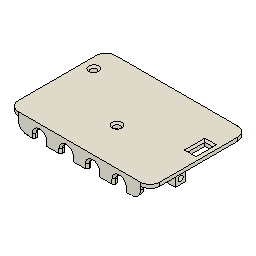
transmitter_assembly (Autodesk Fusion 360 archive; units mm, degrees)
design "transmitter_top_cover"
Autodesk Fusion 360 part; units mm, degrees
note: some values were not read from the file. Chosen so that the rebuilt part matches the saved one: which face or edge a step refers to. Set by a fixed rule: which sketch regions a step uses.
imported_body "Derived Base Feature1" makes body 1 makes body 2
imported_body "Derived Base Feature2" makes body 3 makes body 4
imported_body "Derived Base Feature3" makes body 5
imported_body "Derived Base Feature4" makes body 6
imported_body "Derived Base Feature5" makes body 7
imported_body "Derived Base Feature6" makes body 8
imported_body "Derived Base Feature7" makes body 9
imported_body "Derived Base Feature8" makes body 10
imported_body "Derived Base Feature9" makes body 11
imported_body "Derived Base Feature10" makes body 12
imported_body "Derived Base Feature11" makes body 13
imported_body "Derived Base Feature12" makes body 14
imported_body "Derived Base Feature13" makes body 15
sketch "Sketch1" plane through (0, 0, 0) normal (0, 1, 0) x (1, 0, 0)
  line L0 (34.5, 27.5) -> (-34.5, 27.5)
  line L1 (-40, 22) -> (-40, -22)
  line L2 (-34.5, -27.5) -> (34.5, -27.5)
  line L3 (40, -22) -> (40, 22)
  line L4 (40, 27.5) -> (-40, -27.5) construction
  line L5 (-40, 27.5) -> (40, -27.5) construction
  arc A0 (-34.5, 27.5) -> (-40, 22) centre (-34.5, 22) ccw
  arc A1 (40, 22) -> (34.5, 27.5) centre (34.5, 22) ccw
  arc A2 (34.5, -27.5) -> (40, -22) centre (34.5, -22) ccw
  arc A3 (-40, -22) -> (-34.5, -27.5) centre (-34.5, -22) ccw
  dimension "d1" = 80
  dimension "d2" = 55
  dimension "d3" = 5.5
  constraint horizontal L0
  constraint perpendicular L0 L1
  constraint parallel L0 L2
  constraint parallel L1 L3
  constraint coincident L4 origin
  constraint coincident L5 origin
  constraint coincident L5.start L1
  constraint coincident L5.start L0
  constraint tangent L1 A0
  constraint tangent L0 A0
  constraint coincident L4.start L0
  constraint coincident L4.start L3
  constraint tangent L0 A1
  constraint tangent L3 A1
  constraint coincident L5.end L3
  constraint coincident L5.end L2
  constraint tangent L3 A2
  constraint tangent L2 A2
  constraint equal A1 A2
  constraint coincident L4.end L2
  constraint coincident L4.end L1
  constraint tangent L2 A3
  constraint tangent L1 A3
  constraint equal A1 A3
  constraint equal A0 A1
  measures "d1" distance of L4.end L5.end
  measures "d2" distance of L5.start L4.end
  measures "d3" radius of A0
extrude "Extrude1" add sketch "Sketch1" against normal blind 2 separate body makes body 16
sketch "Sketch2" plane through (0, -2, 0) normal (0, -1, 0) x (1, 0, 0)
  arc A0 (-34.5, 27.5) -> (-40, 22) centre (-34.5, 22) ccw
  line L0 (-40, 22) -> (-40, -22)
  arc A1 (-40, -22) -> (-34.5, -27.5) centre (-34.5, -22) ccw
  line L1 (-34.5, -27.5) -> (34.5, -27.5)
  arc A2 (34.5, -27.5) -> (40, -22) centre (34.5, -22) ccw
  line L2 (40, -22) -> (40, 22)
  arc A3 (40, 22) -> (34.5, 27.5) centre (34.5, 22) ccw
  line L3 (34.5, 27.5) -> (-34.5, 27.5)
  line L4 (34.5, 25.5) -> (-34.5, 25.5)
  line L5 (-38, 22) -> (-38, -22)
  line L6 (-34.5, -25.5) -> (34.5, -25.5)
  line L7 (38, -22) -> (38, 22)
  line L8 (38, 25.5) -> (-38, -25.5) construction
  line L9 (-38, 25.5) -> (38, -25.5) construction
  arc A4 (-34.5, 25.5) -> (-38, 22) centre (-34.5, 22) ccw
  arc A5 (38, 22) -> (34.5, 25.5) centre (34.5, 22) ccw
  arc A6 (34.5, -25.5) -> (38, -22) centre (34.5, -22) ccw
  arc A7 (-38, -22) -> (-34.5, -25.5) centre (-34.5, -22) ccw
  dimension "d7" = 76
  dimension "d8" = 51
  dimension "d9" = 3.5
  constraint horizontal L4
  constraint perpendicular L4 L5
  constraint parallel L4 L6
  constraint parallel L5 L7
  constraint coincident L8 origin
  constraint coincident L9 origin
  constraint coincident L9.start L5
  constraint coincident L9.start L4
  constraint tangent L5 A4
  constraint tangent L4 A4
  constraint coincident L8.start L4
  constraint coincident L8.start L7
  constraint tangent L4 A5
  constraint tangent L7 A5
  constraint coincident L9.end L7
  constraint coincident L9.end L6
  constraint tangent L7 A6
  constraint tangent L6 A6
  constraint equal A5 A6
  constraint coincident L8.end L6
  constraint coincident L8.end L5
  constraint tangent L6 A7
  constraint tangent L5 A7
  constraint equal A5 A7
  constraint equal A4 A5
  measures "d7" distance of L8.end L9.end
  measures "d8" distance of L9.start L8.end
  measures "d9" radius of A4
extrude "Extrude2" add sketch "Sketch2" along normal blind 1 contours L4 L5 L6 L7 A4 A5 A6 A7 bodies 16
sketch "Sketch3" plane through (0, 0, -27.5) normal (0, 0, -1) x (-1, 0, 0)
  line L0 (34.5, 0) -> (-34.5, 0)
  line L1 (-34.5, 0) -> (-34.5, -2)
  line L2 (-34.5, -2) -> (34.5, -2)
  line L3 (34.5, -2) -> (34.5, 0)
  line L4 (-34.5, 0) -> (34.5, 0)
  line L5 (34.5, 0) -> (34.5, -4)
  line L6 (29.5, -9) -> (-29.5, -9)
  line L7 (-34.5, -4) -> (-34.5, 0)
  arc A0 (29.5, -9) -> (34.5, -4) centre (29.5, -4) ccw
  arc A1 (-34.5, -4) -> (-29.5, -9) centre (-29.5, -4) ccw
  point P0 (-34.5, -9)
  dimension "d13" = 9
  dimension "d14" = 5
  constraint horizontal L4
  constraint vertical L5
  constraint horizontal L6
  constraint vertical L7
  constraint coincident L0.end L1.start
  constraint coincident L0.start L3.end
  constraint tangent L5 A0
  constraint tangent L6 A0
  constraint coincident P0 L6
  constraint coincident P0 L7
  constraint tangent L6 A1
  constraint tangent L7 A1
  constraint equal A0 A1
  measures "d13" distance of L0.end P0
  measures "d14" radius of A0
extrude "Extrude3" add sketch "Sketch3" against normal blind 2 bodies 16
mirror "Mirror1" about plane through (0, 0, 0) normal (0, 0, 1) of "Extrude3"
sketch "Sketch4" plane through (0, 0, -27.5) normal (0, 0, -1) x (-1, 0, 0)
  line L0 (34.5, 0) -> (-34.5, 0)
  line L1 (-34.5, 0) -> (-34.5, -2)
  line L2 (-34.5, -2) -> (-34.5, -4)
  arc A0 (-34.5, -4) -> (-29.5, -9) centre (-29.5, -4) ccw
  line L3 (-29.5, -9) -> (29.5, -9)
  arc A1 (29.5, -9) -> (34.5, -4) centre (29.5, -4) ccw
  line L4 (34.5, -4) -> (34.5, -2)
  line L5 (34.5, -2) -> (34.5, 0)
  line L6 (24.8, -5.105) -> (20.2, -5.105)
  line L7 (20.2, -5.105) -> (20.2, -9)
  line L8 (20.2, -9) -> (24.8, -9)
  line L9 (24.8, -9) -> (24.8, -5.105)
  line L10 (5.03, -9) -> (13.97, -9)
  line L11 (13.97, -9) -> (13.97, -7.23)
  line L12 (12.69, -5.95) -> (6.31, -5.95)
  line L13 (5.03, -7.23) -> (5.03, -9)
  line L14 (5.03, -9) -> (13.97, -5.95) construction
  line L15 (13.97, -9) -> (5.03, -5.95) construction
  arc A2 (13.97, -7.23) -> (12.69, -5.95) centre (12.69, -7.23) ccw
  arc A3 (6.31, -5.95) -> (5.03, -7.23) centre (6.31, -7.23) ccw
  line L16 (0, -9) -> (37.5, -9) construction
  line L17 (24.8, -9) -> (20.2, -5.105) construction
  line L18 (20.2, -9) -> (24.8, -5.105) construction
  point P0 (9.5, -7.475)
  point P1 (22.5, -7.0525)
  dimension "d83" = 8.94
  dimension "d84" = 3.05
  dimension "d85" = 1.28
  dimension "d87" = 4.6
  dimension "d88" = 3.895
  dimension "d119" = 37.5
  dimension "d120" = 28
  dimension "d121" = 15
  constraint horizontal L6
  constraint vertical L7
  constraint horizontal L8
  constraint vertical L9
  constraint coincident L3 L7.end
  constraint horizontal L10
  constraint perpendicular L10 L11
  constraint parallel L10 L12
  constraint parallel L11 L13
  constraint coincident L14 P0
  constraint coincident L15 P0
  constraint coincident L14.end L12
  constraint coincident L14.end L11
  constraint tangent L12 A2
  constraint tangent L11 A2
  constraint coincident L15.end L13
  constraint coincident L15.end L12
  constraint tangent L13 A3
  constraint tangent L12 A3
  constraint equal A2 A3
  constraint coincident L3 L10.end
  constraint midpoint L3 L16.start
  constraint perpendicular L13 L16
  constraint coincident L18 P1
  constraint coincident L17 P1
  measures "d83" distance of L14.end L15.end
  measures "d84" distance of L10.end L14.end
  measures "d85" radius of A2
  measures "d87" distance of L6.start L6.end
  measures "d88" distance of L6.start L8.end
  measures "d119" distance of L16.start L16.end
  measures "d120" horizontal distance of P0 L16.end
  measures "d121" horizontal distance of L16.end P1
extrude "Extrude4" cut sketch "Sketch4" against normal up to surface (2 mm away) contours L3 L6 L7 L8 L9 | L3 L10 L11 L12 L13 A2 A3 bodies 16
sketch "Sketch10" plane through (0, 0, 27.5) normal (0, 0, 1) x (1, 0, 0)
  line L0 (34.5, 0) -> (-34.5, 0)
  line L1 (-34.5, 0) -> (-34.5, -2)
  line L2 (-34.5, -2) -> (-34.5, -4)
  arc A0 (-34.5, -4) -> (-29.5, -9) centre (-29.5, -4) ccw
  line L3 (-29.5, -9) -> (29.5, -9)
  arc A1 (29.5, -9) -> (34.5, -4) centre (29.5, -4) ccw
  line L4 (34.5, -4) -> (34.5, -2)
  line L5 (34.5, -2) -> (34.5, 0)
  circle A2 centre (-22.5, -6.5) radius 3.05
  circle A3 centre (-7.5, -6.5) radius 3.05
  circle A4 centre (7.5, -6.5) radius 3.05
  circle A5 centre (22.5, -6.5) radius 3.05
  line L6 (-22.5, -6.5) -> (22.5, -6.5) construction
  line L7 (0, 0) -> (0, -9) construction
  line L8 (-25.55, -6.5) -> (-25.55, -9)
  line L9 (-19.45, -6.5) -> (-19.45, -9)
  line L10 (-10.55, -6.5) -> (-10.55, -9)
  line L11 (-4.45, -6.5) -> (-4.45, -9)
  line L12 (4.45, -6.5) -> (4.45, -9)
  line L13 (10.55, -6.5) -> (10.55, -9)
  line L14 (19.45, -6.5) -> (19.45, -9)
  line L15 (25.55, -6.5) -> (25.55, -9)
  point P0 (0, -6.5)
  dimension "d92" = 15
  dimension "d93" = 0
  dimension "d96" = 6.1
  dimension "d97" = 2.5
  constraint coincident A2.centre L6.start
  constraint coincident A5.centre L6.end
  constraint coincident L7.start origin
  constraint midpoint L3 L7.end
  constraint midpoint L6 P0
  constraint coincident L7 P0
  constraint coincident A2 L8.start
  constraint coincident L3 L8.end
  constraint perpendicular L3 L8
  constraint tangent A2 L8
  constraint coincident A2 L9.start
  constraint coincident L3 L9.end
  constraint perpendicular L3 L9
  constraint tangent A2 L9
  measures "d96" diameter of A2
  measures "d97" distance of L3 A2.centre
extrude "Extrude10" cut sketch "Sketch10" against normal blind 2 contours L3 A5 L15 | L3 A2 L8 | L3 A5 | L3 A2 | L3 A5 L14 | L3 A2 L9 | L3 A4 L13 | L3 A3 L10 | L3 A4 | L3 A3 | L3 A4 L12 | L3 A3 L11 picked at (23.3012, -7.8261) picked at (-23.3086, -6.3422) picked at (8.1001, -5.2539) picked at (-7.5633, -5.6506) bodies 16
sketch "Sketch5" plane through (0, 0, 0) normal (0, 1, 0) x (-1, 0, 0)
  arc A0 (34.5, -27.5) -> (40, -22) centre (34.5, -22) ccw
  line L0 (40, -22) -> (40, 22)
  arc A1 (40, 22) -> (34.5, 27.5) centre (34.5, 22) ccw
  line L1 (34.5, 27.5) -> (-34.5, 27.5)
  arc A2 (-34.5, 27.5) -> (-40, 22) centre (-34.5, 22) ccw
  line L2 (-40, 22) -> (-40, -22)
  arc A3 (-40, -22) -> (-34.5, -27.5) centre (-34.5, -22) ccw
  line L3 (-34.5, -27.5) -> (34.5, -27.5)
  circle A4 centre (42.5, -18) radius 1.5
  circle A5 centre (42.5, -18) radius 1.5
  circle A6 centre (40, 15.27) radius 1.5
  circle A7 centre (30, 15.27) radius 1.5
  circle A8 centre (20, 15.27) radius 1.5
  circle A9 centre (10, 15.27) radius 1.5
  circle A10 centre (-10, 15.27) radius 1.5
  circle A11 centre (-20, 15.27) radius 1.5
  circle A12 centre (-40, 15.27) radius 1.5
  circle A13 centre (-30, 15.27) radius 1.5
  line L4 (-48.016, -4.69) -> (-48.27, -4.944)
  line L5 (-48.27, -4.944) -> (-48.27, -6.976)
  line L6 (-48.27, -6.976) -> (-48.016, -7.23)
  line L7 (-48.016, -7.23) -> (-48.27, -7.484)
  line L8 (-48.27, -7.484) -> (-48.27, -9.516)
  line L9 (-48.27, -9.516) -> (-48.016, -9.77)
  line L10 (-48.016, -9.77) -> (-48.27, -10.024)
  line L11 (-48.27, -10.024) -> (-48.27, -12.056)
  line L12 (-48.27, -12.056) -> (-48.016, -12.31)
  line L13 (-48.016, -12.31) -> (-45.984, -12.31)
  line L14 (-45.984, -12.31) -> (-45.73, -12.056)
  line L15 (-45.73, -12.056) -> (-45.73, -10.024)
  line L16 (-45.73, -10.024) -> (-45.984, -9.77)
  line L17 (-45.984, -9.77) -> (-45.73, -9.516)
  line L18 (-45.73, -9.516) -> (-45.73, -7.484)
  line L19 (-45.73, -7.484) -> (-45.984, -7.23)
  line L20 (-45.984, -7.23) -> (-45.73, -6.976)
  line L21 (-45.73, -6.976) -> (-45.73, -4.944)
  line L22 (-45.73, -4.944) -> (-45.984, -4.69)
  line L23 (-45.984, -4.69) -> (-48.016, -4.69)
  line L24 (-46.68, -5.64) -> (-46.68, -6.28)
  line L25 (-46.68, -6.28) -> (-47.32, -6.28)
  line L26 (-47.32, -6.28) -> (-47.32, -5.64)
  line L27 (-47.32, -5.64) -> (-46.68, -5.64)
  line L28 (-46.68, -8.82) -> (-47.32, -8.82)
  line L29 (-47.32, -8.82) -> (-47.32, -8.18)
  line L30 (-47.32, -8.18) -> (-46.68, -8.18)
  line L31 (-46.68, -8.18) -> (-46.68, -8.82)
  line L32 (-47.32, -10.72) -> (-46.68, -10.72)
  line L33 (-46.68, -10.72) -> (-46.68, -11.36)
  line L34 (-46.68, -11.36) -> (-47.32, -11.36)
  line L35 (-47.32, -11.36) -> (-47.32, -10.72)
  line L36 (-49.27, -13.31) -> (-44.73, -13.31)
  line L37 (-44.73, -13.31) -> (-44.73, -3.69)
  line L38 (-44.73, -3.69) -> (-49.27, -3.69)
  line L39 (-49.27, -3.69) -> (-49.27, -13.31)
  line L40 (-49.27, -13.31) -> (-44.73, -3.69) construction
  line L41 (-44.73, -13.31) -> (-49.27, -3.69) construction
  circle A14 centre (-40, 15.27) radius 1.75
  circle A15 centre (-30, 15.27) radius 1.75
  circle A16 centre (-20, 15.27) radius 1.75
  circle A17 centre (-10, 15.27) radius 1.75
  circle A18 centre (10, 15.27) radius 1.75
  circle A19 centre (20, 15.27) radius 1.75
  circle A20 centre (30, 15.27) radius 1.75
  circle A21 centre (40, 15.27) radius 1.75
  point P0 (-47, -8.5)
  dimension "d22" = 1
  dimension "d23" = 1
  dimension "d24" = 1
  dimension "d25" = 1
  dimension "d69" = 0.25
  dimension "d72" = 80
  dimension "d73" = 0
  constraint horizontal L36
  constraint perpendicular L36 L37
  constraint parallel L36 L38
  constraint parallel L37 L39
  constraint coincident L40 P0
  constraint coincident L41 P0
  measures "d22" distance of L13 L36
  measures "d23" distance of L15 L37
  measures "d24" distance of L23 L38
  measures "d25" distance of L8 L39
extrude "Extrude5" [suppressed]
sketch "Sketch6" plane through (0, -3, 0) normal (0, -1, 0) x (1, 0, 0)
  arc A0 (-38, -22) -> (-34.5, -25.5) centre (-34.5, -22) ccw
  line L0 (-34.5, -25.5) -> (34.5, -25.5)
  arc A1 (34.5, -25.5) -> (38, -22) centre (34.5, -22) ccw
  line L1 (38, -22) -> (38, 22)
  arc A2 (38, 22) -> (34.5, 25.5) centre (34.5, 22) ccw
  line L2 (34.5, 25.5) -> (-34.5, 25.5)
  arc A3 (-34.5, 25.5) -> (-38, 22) centre (-34.5, 22) ccw
  line L3 (-38, 22) -> (-38, -22)
  circle A4 centre (-40, 15.27) radius 2.5
  circle A5 centre (-30, 15.27) radius 2.5
  circle A6 centre (-20, 15.27) radius 2.5
  circle A7 centre (-10, 15.27) radius 2.5
  circle A8 centre (10, 15.27) radius 2.5
  circle A9 centre (20, 15.27) radius 2.5
  circle A10 centre (30, 15.27) radius 2.5
  circle A11 centre (40, 15.27) radius 2.5
  circle A12 centre (-42.5, -18) radius 2.5
  circle A13 centre (-40, 15.27) radius 3.5
  circle A14 centre (-30, 15.27) radius 3.5
  circle A15 centre (-20, 15.27) radius 3.5
  circle A16 centre (-10, 15.27) radius 3.5
  circle A17 centre (10, 15.27) radius 3.5
  circle A18 centre (20, 15.27) radius 3.5
  circle A19 centre (30, 15.27) radius 3.5
  circle A20 centre (40, 15.27) radius 3.5
  circle A21 centre (-42.5, -18) radius 3
  circle A22 centre (-10, 15.27) radius 1.75
  circle A23 centre (10, 15.27) radius 1.75
  circle A24 centre (-20, 15.27) radius 1.75
  circle A25 centre (20, 15.27) radius 1.75
  circle A26 centre (30, 15.27) radius 1.75
  circle A27 centre (-30, 15.27) radius 1.75
  dimension "d35" = 5
  dimension "d36" = 5
  dimension "d44" = 7
  dimension "d45" = 6
  constraint concentric A4 A13
  constraint concentric A5 A14
  constraint concentric A6 A15
  constraint concentric A7 A16
  constraint concentric A8 A17
  constraint concentric A9 A18
  constraint concentric A11 A20
  constraint concentric A12 A21
  constraint equal A10 A11
  constraint equal A9 A10
  constraint equal A8 A9
  constraint equal A7 A8
  constraint equal A6 A7
  constraint equal A5 A6
  constraint equal A4 A5
  constraint equal A19 A20
  constraint equal A18 A19
  constraint equal A17 A18
  constraint equal A16 A17
  constraint equal A15 A16
  constraint equal A14 A15
  constraint equal A13 A14
  measures "d35" diameter of A11
  measures "d36" diameter of A12
  measures "d44" diameter of A20
  measures "d45" diameter of A21
extrude "Extrude6" [suppressed]
sketch "Sketch7" plane through (38, 0, 0) normal (1, 0, 0) x (0, 0, -1)
  line L0 (-22, -2) -> (-22, -3)
  line L1 (-22, -3) -> (22, -3)
  line L2 (22, -3) -> (22, -2)
  line L3 (22, -8.99) -> (-22, -8.99)
  line L4 (-11.225, -3) -> (-5.225, -3)
  line L5 (-5.225, -3) -> (-5.225, -8.99)
  line L6 (-5.225, -8.99) -> (-11.225, -8.99)
  line L7 (-11.225, -8.99) -> (-11.225, -3)
  circle A0 centre (-8.225, -5.995) radius 1.45
  line L8 (22, -2) -> (-22, -2)
  dimension "d48" = 6
  dimension "d49" = 10.775
  dimension "d60" = 2.9
  dimension "d61" = 2.995
  dimension "d62" = 13.775
  constraint horizontal L4
  constraint vertical L5
  constraint horizontal L6
  constraint vertical L7
  constraint coincident L3 L5.end
  constraint coincident L1 L4.start
  measures "d48" distance of L4.start L4.end
  measures "d49" distance of L3.end L7
  measures "d60" diameter of A0
  measures "d61" distance of L3 A0.centre
  measures "d62" horizontal distance of L3.end A0.centre
extrude "Extrude7" add sketch "Sketch7" against normal blind 5 contours L1 L3 L4 L5 L6 L7 bodies 16
sketch "Sketch8" plane through (0, 0, 25.5) normal (0, 0, 1) x (1, 0, 0)
  line L0 (34.5, -2) -> (-34.5, -2)
  line L1 (-34.5, -2) -> (-34.5, -3)
  line L2 (-34.5, -3) -> (34.5, -3)
  line L3 (34.5, -3) -> (34.5, -2)
  line L4 (47, -8.99) -> (-47, -8.99)
  line L5 (-3, -3) -> (3, -3)
  line L6 (3, -3) -> (3, -8.99)
  line L7 (3, -8.99) -> (-3, -8.99)
  line L8 (-3, -8.99) -> (-3, -3)
  circle A0 centre (12.5, -5.995) radius 1.45
  dimension "d52" = 6
  dimension "d53" = 44
  dimension "d63" = 2.9
  dimension "d64" = 47
  dimension "d65" = 2.995
  constraint horizontal L5
  constraint vertical L6
  constraint horizontal L7
  constraint vertical L8
  constraint coincident L2 L5.start
  constraint coincident L4 L6.end
  measures "d52" distance of L5.start L5.end
  measures "d53" distance of L4.end L7.end
  measures "d63" diameter of A0
  measures "d64" distance of L1 A0.centre
  measures "d65" distance of L7 A0.centre
extrude "Extrude8" [suppressed]
sketch "Sketch9" plane through (-38, 0, 0) normal (-1, 0, 0) x (0, 0, 1)
  line L0 (-22, -2) -> (-22, -3)
  line L1 (-22, -3) -> (22, -3)
  line L2 (22, -3) -> (22, -2)
  line L3 (-12, -3) -> (-6, -3)
  line L4 (-6, -3) -> (-6, -8.99)
  line L5 (-6, -8.99) -> (-12, -8.99)
  line L6 (-12, -8.99) -> (-12, -3)
  line L7 (22, -8.99) -> (-22, -8.99)
  circle A0 centre (-9, -5.995) radius 1.45
  line L8 (22, -2) -> (-22, -2)
  dimension "d56" = 6
  dimension "d57" = 10
  dimension "d66" = 2.9
  dimension "d67" = 2.995
  dimension "d68" = 13
  constraint horizontal L3
  constraint vertical L4
  constraint horizontal L5
  constraint vertical L6
  constraint coincident L1 L3.start
  constraint coincident L4.end L7
  measures "d56" distance of L4.end L5.end
  measures "d57" distance of L5.end L7.end
  measures "d66" diameter of A0
  measures "d67" distance of L7 A0.centre
  measures "d68" horizontal distance of L7.end A0.centre
extrude "Extrude9" add sketch "Sketch9" against normal blind 5 contours L1 L3 L4 L5 L6 L7 bodies 16
chamfer "Chamfer1" [suppressed]
chamfer "Chamfer2" distance 1 angle 45 3 edges at (-24.8, -7.0525, -27.5) (-22.5, -5.105, -27.5) (-20.2, -7.0525, -27.5) on bodies 16
chamfer "Chamfer2" distance 1 angle 45 5 edges at (-9.5, -5.95, -27.5) (-5.4049, -6.3249, -27.5) (-5.03, -8.115, -27.5) (-13.97, -8.115, -27.5) (-13.5951, -6.3249, -27.5) on bodies 16
chamfer "Chamfer2" distance 1 angle 45 12 edges at (-22.5, -3.45, 27.5) (-19.45, -7.75, 27.5) (-25.55, -7.75, 27.5) (-7.5, -3.45, 27.5) (-4.45, -7.75, 27.5) (-10.55, -7.75, 27.5) (10.55, -7.75, 27.5) (4.45, -7.75, 27.5) (7.5, -3.45, 27.5) (22.5, -3.45, 27.5) (25.55, -7.75, 27.5) (19.45, -7.75, 27.5) on bodies 16
fillet "Fillet1" [suppressed]
sketch "Sketch11" plane through (0, -3, 0) normal (0, -1, 0) x (1, 0, 0)
  line L0 (-33, -12) -> (-38, -12)
  line L1 (-38, -12) -> (-38, -22)
  arc A0 (-38, -22) -> (-34.5, -25.5) centre (-34.5, -22) ccw
  line L2 (-34.5, -25.5) -> (34.5, -25.5)
  arc A1 (34.5, -25.5) -> (38, -22) centre (34.5, -22) ccw
  line L3 (38, -22) -> (38, 5.225)
  line L4 (38, 5.225) -> (33, 5.225)
  line L5 (33, 5.225) -> (33, 11.225)
  line L6 (33, 11.225) -> (38, 11.225)
  line L7 (38, 11.225) -> (38, 22)
  arc A2 (38, 22) -> (34.5, 25.5) centre (34.5, 22) ccw
  line L8 (34.5, 25.5) -> (-34.5, 25.5)
  arc A3 (-34.5, 25.5) -> (-38, 22) centre (-34.5, 22) ccw
  line L9 (-38, 22) -> (-38, -6)
  line L10 (-38, -6) -> (-33, -6)
  line L11 (-33, -6) -> (-33, -12)
  line L12 (37.5, 25) -> (-37.5, 25) construction
  line L13 (-37.5, 25) -> (-37.5, -25) construction
  line L14 (-37.5, -25) -> (37.5, -25) construction
  line L15 (37.5, -25) -> (37.5, 25) construction
  line L16 (37.5, 25) -> (-37.5, -25) construction
  line L17 (-37.5, 25) -> (37.5, -25) construction
  circle A4 centre (0, 6.27) radius 1.75
  circle A5 centre (0, 6.27) radius 2.5
  circle A6 centre (0, 6.27) radius 3
  line L18 (32.23, -11.27) -> (36.77, -11.27)
  line L19 (36.77, -11.27) -> (36.77, -1.65)
  line L20 (36.77, -1.65) -> (32.23, -1.65)
  line L21 (32.23, -1.65) -> (32.23, -11.27)
  line L22 (32.23, -11.27) -> (36.77, -1.65) construction
  line L23 (36.77, -11.27) -> (32.23, -1.65) construction
  circle A7 centre (-34.23, -14.825) radius 1.75
  circle A8 centre (-34.23, -14.825) radius 2.5
  circle A9 centre (-34.23, -14.825) radius 3
  point P0 (34.5, -6.46)
  dimension "d99" = 75
  dimension "d100" = 50
  dimension "d101" = 37.5
  dimension "d103" = 18.73
  dimension "d104" = 3.5
  dimension "d107" = 5
  dimension "d108" = 6
  dimension "d114" = 3
  dimension "d115" = 18.54
  dimension "d116" = 4.54
  dimension "d117" = 9.62
  dimension "d123" = 3.5
  dimension "d124" = 5
  dimension "d125" = 6
  dimension "d126" = 3.27
  dimension "d131" = 10.175
  constraint horizontal L12
  constraint perpendicular L12 L13
  constraint parallel L12 L14
  constraint parallel L13 L15
  constraint coincident L16 origin
  constraint coincident L17 origin
  constraint concentric A4 A5
  constraint concentric A5 A6
  constraint horizontal L18
  constraint perpendicular L18 L19
  constraint parallel L18 L20
  constraint parallel L19 L21
  constraint coincident L22 P0
  constraint coincident L23 P0
  constraint concentric A7 A8
  constraint concentric A8 A9
  measures "d99" distance of L13.end L14.end
  measures "d100" distance of L12.end L13.end
  measures "d101" horizontal distance of L13.end A4.centre
  measures "d103" distance of L12 A4.centre
  measures "d104" diameter of A4
  measures "d107" diameter of A5
  measures "d108" diameter of A6
  measures "d114" distance of L15 P0
  measures "d115" distance of L14 P0
  measures "d116" distance of L18.start L18.end
  measures "d117" distance of L18.start L20.end
  measures "d123" diameter of A7
  measures "d124" diameter of A8
  measures "d125" diameter of A9
  measures "d126" horizontal distance of L12.end A7.centre
  measures "d131" vertical distance of L13.end A7.centre
extrude "Extrude11" cut sketch "Sketch11" against normal blind 3 contours A4 | L18 L19 L20 L21 | A7 bodies 16
extrude "Extrude12" add sketch "Sketch11" along normal blind 5.99 contours L0 A9 | L0 A9 | A6 bodies 16
chamfer "Chamfer3" distance 1 angle 45 1 edges at (-1.6316, 0, 5.6372) on bodies 16
chamfer "Chamfer3" distance 1 angle 45 4 edges at (34.5, 0, -1.65) (36.77, 0, -6.46) (32.23, 0, -6.46) (34.5, 0, -11.27) on bodies 16
chamfer "Chamfer3" distance 1 angle 45 1 edges at (-35.8616, 0, -15.4578) on bodies 16
fillet "Fillet2" radius 1.5 1 edges at (-2.797, -3, 7.3548) on bodies 16
fillet "Fillet2" radius 1.5 1 edges at (-34.23, -3, -17.825) on bodies 16
chamfer "Chamfer4" distance 1 angle 45 4 edges at (-35.5, -3, -6) (35.5, -3, 11.225) (33, -3, 8.225) (35.5, -3, 5.225) on bodies 16
hidden bodies 1 2 3 4 5 6 7 8 9 10 11 12 13 14 15
equation "d119 = ( 75 / 2 ) * 1 mm"
named bodies: "Body1 (Context1)", "Body3 (Context1)", "Body18 (Context1)", "Body36 (Context1)", "Body1 (1) (Context1)", "Body1 (2) (Context1)", "Body1 (3) (Context1)", "Body1 (4) (Context1)", "Body1 (5) (Context1)", "Body1 (6) (Context1)", "Body1 (7) (Context1)", "Body1 (8) (Context1)", "Body1 (9) (Context1)", "Body1 (10) (Context1)", "Body1 (11) (Context1)"
